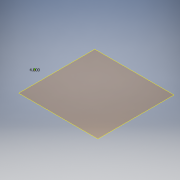
# Autodesk Inventor part: fonl
Saved by Autodesk Inventor 2019 (Build 230136000, 136)
## iProperties
Created: 2019-11-25
Part Number: fonl
Material: Generic
Document SubType Name: Modeling
Designer: Administrator
Density: 1 g/cm^3
Appearance: Default
Author: Administrator
Autodesk Inventor part; units mm, degrees
ref_plane "YZ Plane" through (0, 0, 0) normal (1, 0, 0) x (0, 1, 0)
ref_plane "XZ Plane" through (0, 0, 0) normal (0, 1, 0) x (-1, 0, 0)
ref_plane "XY Plane" through (0, 0, 0) normal (0, 0, 1) x (1, 0, 0)
ref_plane "Work Plane1" through (7940.0938, -7568.4771, -3491.6601) normal (0, 1, 0) x (-1, 0, 0)
sketch "Sketch1" plane through (7940.0938, -7568.4771, -3491.6601) normal (0, 1, 0) x (-1, 0, 0)
  circle A0 centre (7508.1301, 1426.6625) radius 25.4
  point P0 (7940.0938, 3491.6601)
  dimension "d0" = 50.8
  constraints: 1 centre point
  measures "d0" diameter of A0
sketch3d "3D Sketch1"
ref_plane "Work Plane2" through (435.6654, -7466.9445, -2064.9976) normal (0.0364335, 0.9993361, 0) x (-0.9993361, 0.0364335, 0)
sketch "Sketch2" plane through (435.6654, -7466.9445, -2064.9976) normal (0.0364335, 0.9993361, 0) x (-0.9993361, 0.0364335, 0)
  circle A0 centre (0, 0) radius 63.5
  point P0 (707.4228, 2064.9976)
  dimension "d2" = 127
  constraints: 1 centre point
  measures "d2" diameter of A0
loft "Loft1" add profiles "Sketch2", "Sketch1"
shell "Shell1" thickness 2.54 removed faces 2 at (442.5685, -7467.1962, -2046.3452) at (423.819, -7568.4771, -2058.4346)
body "Solid1"
